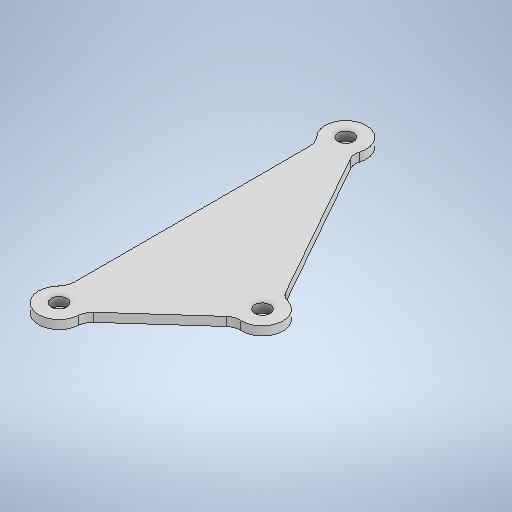
# Autodesk Inventor part: A2P2
Saved by Autodesk Inventor 2025.2 (Build 292293000, 293)
## iProperties
Created: 2025-05-22
Part Number: A2P2
Material: Generic
Document SubType Name: Sheet Metal
Designer: Admin
Density: 1 g/cm^3
Sheet Metal Rule: Default
Appearance: Default
Author: Admin
Autodesk Inventor part; units mm, degrees
ref_plane "YZ Plane" through (0, 0, 0) normal (1, 0, 0) x (0, 1, 0)
ref_plane "XZ Plane" through (0, 0, 0) normal (0, 1, 0) x (-1, 0, 0)
ref_plane "XY Plane" through (0, 0, 0) normal (0, 0, 1) x (1, 0, 0)
sketch "Sketch1" plane through (0, 0, 0) normal (0, 1, 0) x (-1, 0, 0)
  circle A0 centre (0, 0) radius 4
  line L0 (2, -5) -> (2, -50.743)
  line L1 (-2, -7.4505) -> (-2, -43.9092)
  circle A1 centre (0, -55.743) radius 4
  circle A2 centre (-20.8381, -18.7022) radius 4
  line L2 (-4.2089, -6.4649) -> (-16.0918, -17.1298)
  line L3 (-4.9461, -1.7517) -> (-18.5639, -13.9737)
  line L4 (-16.8482, -21.7155) -> (-4.0591, -44.4487)
  line L5 (-20.3344, -23.6767) -> (-3.99, -52.7297)
  arc A3 (2.8966, -2.7586) -> (2, -5) centre (5.25, -5) ccw
  arc A4 (2, -50.743) -> (2.8966, -52.9844) centre (5.25, -50.743) ccw
  arc A5 (-4.9461, -1.7517) -> (-3.9934, 0.2289) centre (-6.8717, 0.3939) ccw
  arc A6 (-20.6355, -14.7073) -> (-18.5639, -13.9737) centre (-20.4894, -11.8283) ccw
  line L6 (0, 0) -> (-20.8381, -18.7022) construction
  line L7 (-20.8381, -18.7022) -> (0, -55.743) construction
  arc A7 (-16.0918, -17.1298) -> (-16.8387, -18.7675) centre (-14.589, -18.8043) ccw
  arc A8 (-17.0295, -19.9247) -> (-16.8482, -21.7155) centre (-14.8872, -20.6123) ccw
  arc A9 (-2, -7.4505) -> (-4.2089, -6.4649) centre (-3.3243, -7.4505) ccw
  arc A10 (-4.0591, -44.4487) -> (-2, -43.9092) centre (-3.1002, -43.9092) ccw
  arc A11 (-20.3344, -23.6767) -> (-21.7708, -22.5919) centre (-22.2953, -24.7799) ccw
  arc A12 (-3.8086, -54.5205) -> (-3.99, -52.7297) centre (-5.951, -53.8329) ccw
  point P0 (-21.4801, -12.8095)
  dimension "d0" = 8
  dimension "d1" = 8
  dimension "d2" = 8
  dimension "d4" = 42.5
  dimension "d5" = 28
  dimension "d6" = 2
  dimension "d7" = 2
  dimension "d8" = 5
  dimension "d10" = 5
  dimension "d11" = 0
  dimension "d12" = 5.2471
  dimension "d14" = 5.247
  dimension "d15" = 2
  dimension "d16" = 2
  dimension "d17" = 2
  dimension "d18" = 2
  dimension "d19" = 4
  dimension "d20" = 5
  dimension "d21" = 5
  dimension "d22" = 5
  dimension "d23" = 1.1002
  dimension "d24" = 1.3243
  dimension "d38" = 55.743
  constraints: 28 point on circle, 20 tangent, 16 end point, 13 centre point, 4 parallel, 2 vertical, 1 coincident
  measures "d0" diameter of A0
  measures "d1" diameter of A1
  measures "d2" diameter of A2
  measures "d4" distance of L6.end L7.end
  measures "d5" distance of point (0, 0) L6.end
  measures "d6" horizontal distance of point (0, 0) L0.start
  measures "d7" horizontal distance of point (0, 0) L1.start
  measures "d8" vertical distance of point (0, 0) L0.start
  measures "d10" vertical distance of L7.end L0.end
  measures "d11" horizontal distance of L7.end point (0, 0)
  measures "d12" distance of L3.start point (0, 0)
  measures "d14" distance of L6.end L3.end
  measures "d15" distance from line of L6 L3.start
  measures "d16" distance from line of L6 L2.end
  measures "d17" distance from line of L7 L4.end
  measures "d18" distance from line of L7 L5.end
  measures "d19" distance of L4.start L5.start
  measures "d20" distance of L5.end L7.end
  measures "d21" distance of L6.end L4.start
  measures "d22" distance of L6.end L2.end
  measures "d23" distance from line of L4 A10.centre
  measures "d24" radius of A9
  measures "d38" distance of point (0, 0) L7.end
extrude "Extrusion1" add sketch "Sketch1" along normal blind 4 contours A0 | A2 | A1
extrude "Extrusion2" add sketch "Sketch1" along normal blind 1.7 contours A0 A3 L0 A4 A1 A12 L5 A11 A2 A8 L4 A10 L1 A9 L2 A7 A6 L3 A5 | A7 L2 A9 L1 A10 L4 A8 A2
sketch "Sketch2" plane through (0, 4, 0) normal (0, 1, 0) x (1, 0, 0)
  circle A0 centre (0, 0) radius 4 projected
  circle A1 centre (0, 0) radius 1.5
  circle A2 centre (20.8381, 18.7022) radius 4 projected
  circle A3 centre (20.8381, 18.7022) radius 1.5
  circle A4 centre (0, 55.743) radius 1.5
  circle A5 centre (0, 55.743) radius 4 projected
  dimension "d29" = 3
  dimension "d30" = 3
  dimension "d31" = 3
  dimension "d36" = 0
  constraints: 3 centre point, 2 coincident
  measures "d29" diameter of A1
  measures "d30" diameter of A4
  measures "d31" diameter of A3
  measures "d36" distance of A5.centre A4.centre
extrude "Extrusion3" cut sketch "Sketch2" against normal blind 4 contours A1 | A3 | A4
sketch "Sketch3" plane through (-2, 0, -50.743) normal (-1, 0, 0) x (0, 0, 1)
  line L0 (60.4555, 1.7) -> (-13.4083, 1.7)
  line L1 (-13.4083, 1.7) -> (-13.4083, 27.1644)
  line L2 (-13.4083, 27.1644) -> (60.4555, 27.1644)
  line L3 (60.4555, 27.1644) -> (60.4555, 1.7)
  point P0 (50.743, 0)
  constraints: 8 end point, 2 parallel, 1 horizontal, 1 perpendicular
extrude "Extrusion4" cut sketch "Sketch3" along normal mid plane 100
equation "\"BendRadius\" = Thickness"
equation "\"BendReliefWidth\" = Thickness"
equation "\"BendReliefDepth\" = 0.5 * Thickness"
equation "\"CornerReliefSize\" = 4 * Thickness"
equation "\"MinimumRemnant\" = 2 * Thickness"
equation "\"TransitionRadius\" = BendRadius"
equation "\"JacobiRadiusSize\" = BendRadius"
equation "\"GapSize\" = Thickness"
equation "\"Thickness\" = 3.048"
body "Solid1"
